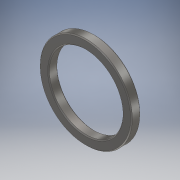
# Autodesk Inventor part: bearing100-80-10
Saved by Autodesk Inventor 2018 (Build 220112000, 112)
## iProperties
Created: 2025-02-24
Part Number: bearing100-80-10
Material: Steel, Galvanized
Document SubType Name: Modeling
Designer: neo
Density: 7.85 g/cm^3
Appearance: Galvanized
Author: neo
Autodesk Inventor part; units mm, degrees
ref_plane "YZ Plane" through (0, 0, 0) normal (1, 0, 0) x (0, 1, 0)
ref_plane "XZ Plane" through (0, 0, 0) normal (0, 1, 0) x (-1, 0, 0)
ref_plane "XY Plane" through (0, 0, 0) normal (0, 0, 1) x (1, 0, 0)
sketch "Sketch1" plane through (0, 0, 0) normal (1, 0, 0) x (0, 1, 0)
  line L0 (15.4505, 45.3153) -> (5.4505, 45.3153)
  line L1 (5.4505, 45.3153) -> (5.4505, 35.3153)
  line L2 (5.4505, 35.3153) -> (15.4505, 35.3153)
  line L3 (15.4505, 35.3153) -> (15.4505, 45.3153)
  line L4 (29.1713, -4.6847) -> (-18.7008, -4.6847)
  point P0 (0, 0)
  dimension "d0" = 10
  dimension "d1" = 10
  dimension "d3" = 100
  constraints: 10 end point, 2 horizontal, 2 parallel, 1 perpendicular
  measures "d0" distance of L2.end L0.start
  measures "d1" distance of L0.start L0.end
  measures "d3" diameter of L0 L4
revolve "Revolution1" add sketch "Sketch1" angle 360 about axis through (0, 29.1713, -4.6847) along (0, -1, 0)
chamfer "Chamfer1" distance 1 angle 45 4 edges at (0, 15.4505, -54.6847) (0, 5.4505, -54.6847) (0, 15.4505, -44.6847) (0, 5.4505, -44.6847)
body "Solid1"
